Support motor rotor (Autodesk Fusion 360 design; units mm, degrees)
Autodesk Fusion 360 part; units mm, degrees
note: some values were not read from the file. Set by a fixed rule: which sketch regions a step uses.
sketch "Sketch1" plane through (0, 0, 0) normal (0, 0, 1) x (1, 0, 0)
  circle A0 centre (0, 0) radius 12.4
  circle A1 centre (0, 0) radius 13.4
  circle A2 centre (0, 0) radius 1.1
  circle A3 centre (0, 0) radius 15
  circle A4 centre (0, 0) radius 16
  dimension "d1" = 24.8
  dimension "d2" = 1
  dimension "d8" = 2.2
  dimension "d103" = 30
  dimension "d117" = 32
  constraint coincident A0.centre A1.centre
  constraint concentric A0 A2
  measures "d1" diameter of A0
  measures "d8" diameter of A2
  measures "d103" diameter of A3
  measures "d117" diameter of A4
extrude "Extrude1" add sketch "Sketch1" against normal blind 2 contours A0 | A1 | A3 makes body 1
extrude "Extrude2" add sketch "Sketch1" along normal blind 34 contours A1 bodies 1
ref_plane "WorkPlane2" through (0, -15, 0) normal (0, 1, 0) x (0, 0, 1)
sketch "Sketch3" plane through (0, -15, 0) normal (0, 1, 0) x (1, 0, 0)
sketch "Sketch4" plane through (0, -15, 0) normal (0, 1, 0) x (1, 0, 0)
  line L0 (-13.4, -34) -> (13.4, -34)
  line L1 (-8.4, -34) -> (-3.3, -34)
  line L2 (7.8, -34) -> (7.8, -14)
  line L3 (7.8, -14) -> (-8.4, -14)
  line L4 (-8.4, -14) -> (-8.4, -34)
  line L5 (9.2, -77) -> (9.2, -34)
  line L6 (9.2, -34) -> (-15.8, -34)
  line L7 (-15.8, -34) -> (-15.8, -77)
  line L8 (-3.3, -77) -> (-3.3, -34) construction
  line L9 (-8.3, -77) -> (-8.3, -62.0106)
  line L10 (1.7, -77) -> (1.7, -62.0106)
  line L11 (-15.8, -77) -> (-8.3, -77)
  line L12 (1.7, -77) -> (9.2, -77)
  arc A0 (1.7, -62.0106) -> (-8.3, -62.0106) centre (-3.3, -62.0106) ccw
  line L13 (-12.3, -74) -> (5.7, -74) construction
  line L14 (5.7, -74) -> (5.7, -41) construction
  line L15 (5.7, -41) -> (-12.3, -41) construction
  line L16 (-12.3, -41) -> (-12.3, -74) construction
  circle A1 centre (5.7, -41) radius 1.6
  circle A2 centre (-12.3, -41) radius 1.6
  circle A3 centre (-12.3, -74) radius 1.6
  circle A4 centre (5.7, -74) radius 1.6
  line L17 (13.4, 0) -> (-13.4, 0)
  line L18 (9.2, -34) -> (-15.8, -34)
  line L19 (-15.8, -34) -> (-15.8, -14)
  line L20 (-15.8, -14) -> (9.2, -14)
  line L21 (9.2, -14) -> (9.2, -34)
  dimension "d55" = 5
  dimension "d57" = 25
  dimension "d58" = 43
  dimension "d62" = 7.4
  dimension "d64" = 10
  dimension "d66" = 33
  dimension "d67" = 18
  dimension "d69" = 3.5
  dimension "d70" = 3.5
  dimension "d71" = 3.2
  dimension "d72" = 3.2
  dimension "d73" = 3.2
  dimension "d74" = 3.2
  dimension "d76" = 7
  dimension "d85" = 20
  constraint horizontal L1
  constraint vertical L2
  constraint horizontal L3
  constraint vertical L4
  constraint coincident L0 L1.start
  constraint horizontal L11
  constraint vertical L5
  constraint horizontal L6
  constraint vertical L7
  constraint coincident L1.start L6
  constraint midpoint L6 L1.end
  constraint coincident L8 A0.centre
  constraint tangent L9 A0
  constraint perpendicular L9 L11
  constraint coincident L10.start L11
  constraint tangent L10 A0
  constraint perpendicular L10 L11
  constraint collinear L11 L12
  constraint coincident L8.start L11
  constraint horizontal L13
  constraint vertical L14
  constraint horizontal L15
  constraint vertical L16
  constraint coincident L14.end L15.start
  constraint coincident L15.end L16.start
  constraint coincident L13.start L16.end
  constraint coincident L13.end L14.start
  constraint horizontal L18
  constraint vertical L19
  constraint horizontal L20
  constraint vertical L21
  constraint coincident L6.end L7.start
  measures "d55" distance of L0.start L1.start
  measures "d57" distance of L7.end L5.start
  measures "d58" distance of L7.end L6.end
  measures "d62" distance of L1.start L6.end
  measures "d64" diameter of A0
  measures "d66" distance of L13.start L15.end
  measures "d67" distance of L13.start L13.end
  measures "d69" distance of L5 L14.end
  measures "d70" distance of L7 L15.end
  measures "d71" diameter of A1
  measures "d72" diameter of A2
  measures "d73" diameter of A3
  measures "d74" diameter of A4
  measures "d76" distance of L1 L14.end
  measures "d85" distance of L2.start L2.end
extrude "Extrude6" add sketch "Sketch4" against normal blind 2 separate body makes body 2
extrude "Extrude7" add sketch "Sketch4" along normal blind 13 contours L0 L4 L6 L18 L19 L20 | L0 L1 L2 L3 L4 L6 L18 L20 | L0 L2 L6 L18 L20 L21 bodies 1 2
extrude "Extrude9" cut 1 faces at (8.5831, -0.6707, 0) along direction (0, 0, 1) blind 35 on bodies 1 bodies 1
extrude "Extrude10" add 1 faces at (14.4108, -0.7452, 0) along direction (0, 0, 1) blind 34 on bodies 1 bodies 1
fillet "Fillet3" radius 3 2 edges at (9.2, -16, 77) (-15.8, -16, 77) on bodies 1
fillet "Fillet2" radius 12.5 1 edges at (-3.3, -17, 14) on bodies 1
fillet "Fillet6" radius 2.5 1 edges at (9.2, -11.8474, 25.1937) on bodies 1
extrude "Extrude13" add sketch "Sketch1" against normal blind 2 contours A4 bodies 1
sketch "Sketch6" plane through (0, 0, -2) normal (0, 0, -1) x (1, 0, 0)
  line L0 (1.6, -16.8286) -> (-1.6, -16.8286)
  line L1 (-1.6, -16.8286) -> (-1.6, 16.8286)
  line L2 (-1.6, 16.8286) -> (1.6, 16.8286)
  line L3 (1.6, 16.8286) -> (1.6, -16.8286)
  line L4 (1.6, -16.8286) -> (-1.6, 16.8286) construction
  line L5 (-1.6, -16.8286) -> (1.6, 16.8286) construction
  circle A0 centre (0, 0) radius 7.5
  circle A1 centre (0, 0) radius 1.1
  circle A2 centre (0, 0) radius 16
  dimension "d108" = 3.2
  dimension "d111" = 15
  constraint perpendicular L0 L1
  constraint parallel L0 L2
  constraint parallel L1 L3
  constraint horizontal L0
  constraint coincident L4 A0.centre
  constraint coincident L5 A0.centre
  constraint coincident A0.centre A1.centre
  measures "d108" distance of L1.end L2.end
  measures "d111" diameter of A0
extrude "Extrude11" cut sketch "Sketch6" against normal blind 3 contours L1 L3 A0 A2 | L1 L3 A0 A2 bodies 1
fillet "Fillet7" radius 5 1 edges at (-15.8, -2, 24) on bodies 1
sketch "Sketch7" plane through (0, 0, -2) normal (0, 0, -1) x (1, 0, 0)
  circle A0 centre (0, 0) radius 12.4
  line L0 (0, 0) -> (0, -12.4) construction
  line L1 (-10.745, 10.3072) -> (-12.3181, 8.3641)
  arc A1 (-12.3181, 8.3641) -> (-8.802, 8.7342) centre (-10.375, 6.7911) ccw
  arc A2 (-10.375, 6.7911) -> (-10.745, 10.3072) centre (-8.802, 8.7342) ccw
  dimension "d115" = 5
  dimension "d116" = 5
  constraint coincident A0.centre L0.start
  constraint coincident A0 L0.end
  constraint vertical L0
  constraint coincident A0 A1.centre
  constraint coincident A0 A1.end
  constraint tangent L1 A1
  measures "d115" diameter of A1
  measures "d116" diameter of A2
extrude "Extrude12" cut sketch "Sketch7" against normal through all contours A0 L1 A1 A2 bodies 1
copy_body "Body->Comp2" bodies 1 removing the originals makes body 3 in component "Support Motor"
sketch "Sketch1 (2)" plane through (0, 0, 0) normal (0, 0, 1) x (1, 0, 0) in component "Head Motor v3"
  line L0 (-16, -23) -> (16, -23)
  line L1 (16, -23) -> (16, 23)
  line L2 (16, 23) -> (-16, 23)
  line L3 (-16, 23) -> (-16, -23)
  line L4 (-16, -23) -> (16, 23) construction
  line L5 (16, -23) -> (-16, 23) construction
  dimension "d1_1" = 46
  dimension "d2_1" = 32
  constraint perpendicular L0 L1
  constraint parallel L0 L2
  constraint parallel L1 L3
  constraint horizontal L0
  constraint coincident L4 origin
  constraint coincident L5 origin
  measures "d1_1" distance of L0.end L1.end
  measures "d2_1" distance of L1.end L2.end
extrude "Extrude1'" add sketch "Sketch1 (2)" along normal blind 23 separate body makes body 4 in component "Head Motor v3"
sketch "Sketch2" plane through (0, 0, 23) normal (0, 0, 1) x (-1, 0, 0) in component "Head Motor v3"
  line L0 (16, -23) -> (16, 23)
  line L1 (16, 23) -> (-16, 23)
  line L2 (-16, 23) -> (-16, -23)
  line L3 (-16, -23) -> (16, -23)
  line L4 (-9, 16.5) -> (9, 16.5) construction
  line L5 (9, 16.5) -> (9, -16.5) construction
  line L6 (9, -16.5) -> (-9, -16.5) construction
  line L7 (-9, -16.5) -> (-9, 16.5) construction
  line L8 (-9, 16.5) -> (9, -16.5) construction
  line L9 (9, 16.5) -> (-9, -16.5) construction
  circle A0 centre (-9, -16.5) radius 3.5
  circle A1 centre (9, -16.5) radius 3.5
  circle A2 centre (-9, 16.5) radius 3.5
  circle A3 centre (9, 16.5) radius 3.5
  line L10 (0, -23) -> (0, 23) construction
  circle A4 centre (0, -8) radius 3
  circle A5 centre (9, -16.5) radius 1.5
  circle A6 centre (-9, -16.5) radius 1.5
  circle A7 centre (9, 16.5) radius 1.5
  circle A8 centre (-9, 16.5) radius 1.5
  dimension "d5_1" = 33
  dimension "d6_1" = 18
  dimension "d7" = 7
  dimension "d8_1" = 7
  dimension "d9" = 7
  dimension "d10" = 7
  dimension "d13" = 6
  dimension "d14" = 15
  dimension "d34" = 3
  dimension "d35" = 3
  dimension "d36" = 3
  dimension "d37" = 3
  constraint perpendicular L4 L5
  constraint parallel L4 L6
  constraint parallel L5 L7
  constraint horizontal L4
  constraint coincident L8 origin
  constraint coincident L9 origin
  constraint coincident L6.end L7.start
  constraint coincident L5.end L6.start
  constraint coincident L4.start L7.end
  constraint coincident L4.end L5.start
  constraint midpoint L3 L10.start
  constraint midpoint L1 L10.end
  constraint coincident L10 A4.centre
  constraint concentric A1 A5
  constraint concentric A3 A7
  constraint concentric A2 A8
  measures "d5_1" distance of L4.end L5.end
  measures "d6_1" distance of L5.end L6.end
  measures "d7" diameter of A0
  measures "d8_1" diameter of A1
  measures "d9" diameter of A2
  measures "d10" diameter of A3
  measures "d13" diameter of A4
  measures "d14" distance of L3 A4.centre
  measures "d34" diameter of A5
  measures "d35" diameter of A6
  measures "d36" diameter of A7
  measures "d37" diameter of A8
extrude "Extrude2'" add sketch "Sketch2" along normal blind 2 contours A0 | A1 | A2 | A3 bodies 4 in component "Head Motor v3"
extrude "Extrude3" add sketch "Sketch2" along normal blind 19 contours A4 bodies 4 in component "Head Motor v3"
fillet "Fillet1" radius 1 4 faces at (16, -7.6667, 7.6667) (-5.3333, -23, 7.6667) (-16, 7.6667, 7.6667) (5.3333, 23, 7.6667) on bodies 4 in component "Head Motor v3"
fillet "Fillet2'" radius 0.5 1 edges at (-5.7369, -15.2343, 25) 4 faces at (6.1853, 16.7484, 25) (6.1853, -16.2516, 25) (-11.8147, 16.7484, 25) (-11.8147, -16.2516, 25) on bodies 4 in component "Head Motor v3"
fillet "Fillet3'" radius 1 1 faces at (0.5, 8.866, 42) on bodies 4 in component "Head Motor v3"
sketch "Sketch4 (2)" plane through (-3, 23, 11.5) normal (0, 1, 0) x (-1, 0, 0) in component "Head Motor v3"
sketch "Sketch5" plane through (0, -23, 0) normal (0, -1, 0) x (1, 0, 0) in component "Head Motor v3"
  line L0 (-15, 1) -> (15, 1)
  line L1 (15, 1) -> (15, 22)
  line L2 (15, 22) -> (-15, 22)
  line L3 (-15, 22) -> (-15, 1)
  circle A0 centre (3, 10) radius 12
  point P0 (16, 22)
  dimension "d25" = 24
  dimension "d26" = 10
  dimension "d27" = 13
  measures "d25" diameter of A0
  measures "d26" vertical distance of origin A0.centre
  measures "d27" horizontal distance of A0.centre P0
extrude "Extrude5" add sketch "Sketch5" along normal blind 31 contours L0 A0 | L0 A0 bodies 4 in component "Head Motor v3"
sketch "Sketch8" plane through (0, -54, 0) normal (0, -1, 0) x (1, 0, 0) in component "Head Motor v3"
  circle A0 centre (3, 10) radius 12
  circle A1 centre (3, 10) radius 11.8
  dimension "d31" = -0.2
extrude "Extrude6'" cut sketch "Sketch8" against normal blind 1 contours A1 bodies 4 in component "Head Motor v3"
component "Support Motor" placed x (1, 0, 0) y (0, 1, 0) z (0, 0, 1) at (0, 0, 0)
component "Head Motor v3" placed x (1, 0, 0) y (0, 0, 1) z (0, -1, 0) at (-3.3, 10, 57.5)
named bodies: "Support Motor"
